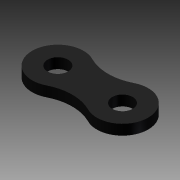
# Autodesk Inventor part: Concha1
Saved by Autodesk Inventor 2011 (Build 150239000, 239)
## iProperties
Created: 2011-08-31
Part Number: Concha1
Document SubType Name: Modeling
Designer: Luis
Density: 1 g/cm^3
Author: Luis
Autodesk Inventor part; units mm, degrees
ref_plane "YZ Plane" through (0, 0, 0) normal (1, 0, 0) x (0, 1, 0)
ref_plane "XZ Plane" through (0, 0, 0) normal (0, 1, 0) x (-1, 0, 0)
ref_plane "XY Plane" through (0, 0, 0) normal (0, 0, 1) x (1, 0, 0)
sketch "Sketch1" plane through (0, 0, 0) normal (0, 0, 1) x (1, 0, 0)
  line L0 (-6.3, 0) -> (6.3, 0) construction
  circle A0 centre (-6.3, 0) radius 2
  circle A1 centre (6.3, 0) radius 2
  arc A2 (-3.9971, 4.4381) -> (-3.9971, -4.4381) centre (-6.3, 0) ccw
  arc A3 (3.9971, -4.4381) -> (3.9971, 4.4381) centre (6.3, 0) ccw
  line L1 (0, 0) -> (0, 3.5) construction
  line L2 (0, 0) -> (0, -3.5) construction
  arc A4 (-3.9971, 4.4381) -> (3.9971, 4.4381) centre (0, 12.4846) ccw
  arc A5 (3.9971, -4.4381) -> (-3.9971, -4.4381) centre (0, -12.4846) ccw
  point P0 (4.1509, 4.5146)
  point P1 (-4.1509, 4.5146)
  point P2 (4.1509, -4.5146)
  point P3 (-4.1509, -4.5146)
  dimension "d0" = 12.6
  dimension "d1" = 4
  dimension "d2" = 4
  dimension "d3" = 10
  dimension "d4" = 10
  dimension "d5" = 3.5
  constraints: 11 point on circle, 6 centre point, 6 coincident, 6 end point, 4 symmetric about line, 1 horizontal, 1 midpoint, 1 perpendicular, 1 other
  measures "d0" distance of L0.start L0.end
  measures "d1" diameter of A0
  measures "d2" diameter of A1
  measures "d3" diameter of A2
  measures "d4" diameter of A3
  measures "d5" distance of L1.start L1.end
extrude "Extrusion1" add sketch "Sketch1" along normal blind 2
body "Solid1"
